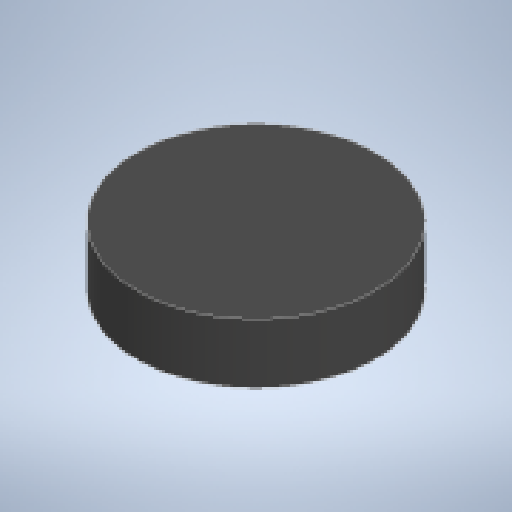
# Autodesk Inventor part: Placeholder (Gear - M)
Saved by Autodesk Inventor 2023.2 (Build 272271000, 271)
## iProperties
Created: 2022-08-10
Part Number: Placeholder (Gear - M)
Material: Nylon 6/6
Document SubType Name: Modeling
Designer: Nathan Cai
Density: 1.13 g/cm^3
Appearance: Rubber - Black
Author: Nathan Cai
Autodesk Inventor part; units mm, degrees
ref_plane "YZ Plane" through (0, 0, 0) normal (1, 0, 0) x (0, 1, 0)
ref_plane "XZ Plane" through (0, 0, 0) normal (0, 1, 0) x (-1, 0, 0)
ref_plane "XY Plane" through (0, 0, 0) normal (0, 0, 1) x (1, 0, 0)
sketch "Sketch1" plane through (0, 0, 0) normal (0, 1, 0) x (-1, 0, 0)
  circle A0 centre (0, 0) radius 19.05
  dimension "d0" = 38.1
  constraints: 1 centre point, 1 coincident
  measures "d0" diameter of A0
extrude "Extrusion1" add sketch "Sketch1" along normal blind 9.525
body "Solid1"
